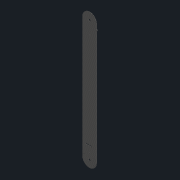
# Autodesk Inventor part: link3-plate1
Saved by Autodesk Inventor 2021 (Build 250183000, 183)
## iProperties
Created: 2021-07-15
Part Number: link3-plate1
Material: CFRP
Document SubType Name: Sheet Metal
Designer: yuta0
Density: 1.43 g/cm^3
Sheet Metal Rule: Default
Appearance: カーボンファイバー
Mass: 67.5813 g
Surface Area: 497.688 cm^2
Volume: 47.2597 cm^3
購入先: カーボン
在庫数: 0.0
Author: yuta0
Autodesk Inventor part; units mm, degrees
ref_plane "YZ Plane" through (0, 0, 0) normal (1, 0, 0) x (0, 1, 0)
ref_plane "XZ Plane" through (0, 0, 0) normal (0, 1, 0) x (-1, 0, 0)
ref_plane "XY Plane" through (0, 0, 0) normal (0, 0, 1) x (1, 0, 0)
sketch "スケッチ1" plane through (0, 0, 0) normal (0, 0, 1) x (1, 0, 0)
  circle A0 centre (0, 0) radius 25
  circle A1 centre (0, 440) radius 25
  line L0 (-25, 0) -> (-25, 440)
  line L1 (25, 440) -> (25, 0)
  dimension "d0" = 50
  dimension "d1" = 50
  dimension "d2" = 440
  measures "d0" diameter of A0
  measures "d1" diameter of A1
  measures "d2" distance of A0.centre A1.centre
extrude "プレート1" add sketch "スケッチ1" along normal blind 2
sketch "スケッチ4" plane through (0, 0, 0) normal (0, 0, -1) x (-1, 0, 0)
  circle A0 centre (0, 0) radius 4
  dimension "d28" = 8
  constraints: 1 centre point, 1 coincident
  measures "d28" diameter of A0
extrude "押し出し1" cut sketch "スケッチ4" against normal blind 10
sketch "スケッチ5" plane through (0, 0, 0) normal (0, 0, -1) x (-1, 0, 0)
  circle A0 centre (0, 0) radius 21
  point P0 (0, 21)
  point P1 (-18.1865, 10.5)
  point P2 (-18.1865, -10.5)
  point P3 (0, -21)
  point P4 (18.1865, -10.5)
  point P5 (18.1865, 10.5)
  dimension "d31" = 42
  dimension "d34" = 360
  constraints: 1 coincident, 1 vertical alignment, 9 other
hole "穴3" at (0, 21, 0) at (18.1865, 10.5, 0) at (18.1865, -10.5, 0) at (0, -21, 0) at (-18.1865, -10.5, 0) at (-18.1865, 10.5, 0) direction (0, 0, 1) diameter 3.2 end through all clearance for "Flat Head Machine Screw" size "M3" standard "Ansi Metric M Profile"
sketch "スケッチ6" plane through (0, 0, 2) normal (0, 0, 1) x (1, 0, 0)
  arc A0 (25, 440) -> (-25, 440) centre (0, 440) ccw projected
  circle A1 centre (0, 440) radius 4
  point P0 (0, 0)
  dimension "d43" = 8
  constraints: 1 centre point, 1 coincident
  measures "d43" diameter of A1
extrude "押し出し2" cut sketch "スケッチ6" against normal blind 10
sketch "スケッチ8" plane through (0, 0, 2) normal (0, 0, 1) x (1, 0, 0)
  arc A0 (25, 440) -> (-25, 440) centre (0, 440) ccw projected
  point P0 (0, 0)
  point P1 (-13, 45)
  point P2 (0, 395)
  point P3 (0, 220)
  dimension "d54" = 45
  dimension "d55" = 220
  dimension "d71" = 45
  dimension "d72" = 13
  constraints: 2 vertical alignment
  measures "d54" distance of A0.centre point (0, 395)
  measures "d55" distance of point (0, 0) point (0, 220)
  measures "d71" vertical distance of point (0, 0) point (-13, 45)
  measures "d72" horizontal distance of point (0, 0) point (-13, 45)
hole "穴4" at (-13, 45, 2) at (0, 395, 2) at (0, 220, 2) direction (0, 0, -1) diameter 4.3 end through all clearance for "Flat Head Machine Screw" size "M4" standard "Ansi Metric M Profile"
sketch "スケッチ10" plane through (0, 0, 2) normal (0, 0, 1) x (1, 0, 0)
  circle A0 centre (7, 45) radius 2.15
  line L0 (7, 45) -> (-13, 45) construction
  line L1 (7, 47.15) -> (-13, 47.15)
  line L2 (-13, 42.85) -> (7, 42.85)
  arc A1 (7, 42.85) -> (7, 47.15) centre (7, 45) ccw
  arc A2 (-13, 47.15) -> (-13, 42.85) centre (-13, 45) ccw
  circle A3 centre (-13, 45) radius 2.15 projected
  point P0 (0, 0)
  point P1 (-3, 45)
  point P2 (7, 47.15)
  point P3 (7, 42.85)
  dimension "d68" = 20
  constraints: 8 end point, 6 tangent, 4 point on circle, 3 centre point, 1 coincident, 1 horizontal, 1 midpoint, 1 parallel
  measures "d68" distance of L0.start L0.end
extrude "押し出し3" cut sketch "スケッチ10" against normal blind 10
sketch "スケッチ11" plane through (0, 0, 2) normal (0, 0, 1) x (1, 0, 0)
  circle A0 centre (25, 420) radius 3
  line L0 (25, 440) -> (25, 0) projected
  circle A1 centre (0, 440) radius 4 projected
  line L1 (22, 425) -> (28, 425)
  line L2 (28, 425) -> (28, 415)
  line L3 (28, 415) -> (22, 415)
  line L4 (22, 415) -> (22, 425)
  line L5 (22, 425) -> (28, 415) construction
  line L6 (28, 425) -> (22, 415) construction
  point P0 (0, 0)
  point P1 (25, 423)
  point P2 (25, 417)
  point P3 (28, 420)
  dimension "d73" = 6
  dimension "d74" = 0
  dimension "d75" = 20
  dimension "d79" = 10
  constraints: 12 end point, 2 midpoint, 2 parallel, 1 centre point, 1 horizontal, 1 perpendicular, 1 tangent
  measures "d73" diameter of A0
  measures "d74" distance from line of L0 A0.centre
  measures "d75" vertical distance of A1.centre A0.centre
  measures "d79" distance of L1.end L2.end
extrude "押し出し4" add sketch "スケッチ11" against normal up to surface (2 mm away) contours A0 L0 | L2 L3 L0 A0 | A0 L0 L1 L2 | L0 A0 | A0 L4 L1 L0 | L0 L3 L4 A0
fillet "コーナーR1" radius 1.5 4 edges at (25, 425, 1) (28, 425, 1) (28, 415, 1) (25, 415, 1)
mirror "ミラー1" about plane through (0, 0, 0) normal (1, 0, 0) of "押し出し4", "コーナーR1"
fillet_without_effect "コーナーR2"
equation "\"d41\" = Thickness"
equation "\"d3\" = Thickness"
equation "\"BendRadius\" = Thickness"
equation "\"BendReliefWidth\" = Thickness"
equation "\"BendReliefDepth\" = 0.5 * Thickness"
equation "\"CornerReliefSize\" = 4 * Thickness"
equation "\"MinimumRemnant\" = 2 * Thickness"
equation "\"TransitionRadius\" = BendRadius"
equation "\"JacobiRadiusSize\" = Thickness"
equation "\"GapSize\" = Thickness"
equation "\"Thickness\" = 2"
